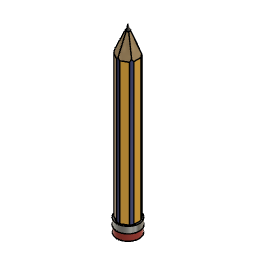
Pencil (Autodesk Fusion 360 design; units mm, degrees)
Autodesk Fusion 360 part; units mm, degrees
sketch "Sketch4" plane through (0, 0, 0) normal (0, 0, 1) x (1, 0, 0)
  line L0 (10, 5.7735) -> (0, 11.547)
  line L1 (0, 11.547) -> (-10, 5.7735)
  line L2 (-10, 5.7735) -> (-10, -5.7735)
  line L3 (-10, -5.7735) -> (0, -11.547)
  line L4 (0, -11.547) -> (10, -5.7735)
  line L5 (10, -5.7735) -> (10, 5.7735)
extrude "Extrude3" add sketch "Sketch4" along normal blind 150
ref_plane "WorkPlane2" through (0, 0, 172) normal (0, 0, 1) x (1, 0, 0)
sketch "Sketch6" plane through (0, 0, 172) normal (0, 0, 1) x (1, 0, 0)
  circle A0 centre (0, 0) radius 2
  constraint coincident A0.centre origin
loft "Loft1" add profiles "Sketch6" section 1 face at (3.3333, 1.9245, 150) section 2
ref_plane "WorkPlane3" through (0, 0, 178) normal (0, 0, 1) x (1, 0, 0)
sketch "Sketch7" plane through (0, 0, 178) normal (0, 0, 1) x (1, 0, 0)
  circle A0 centre (0, 0) radius 0.0005
  dimension "d11" = 0.001
  constraint coincident A0.centre origin
  measures "d11" diameter of A0
loft "Loft2" add section 1 face at (-0.1251, 0.4887, 172) section 2 point at (0, 0, 178)
sketch "Sketch8" plane through (0, 0, 0) normal (0, 0, -1) x (1, 0, 0)
  line L0 (10, -5.7735) -> (10, 5.7735)
  line L1 (10, 5.7735) -> (0, 11.547)
  line L2 (0, 11.547) -> (-10, 5.7735)
  line L3 (-10, 5.7735) -> (-10, -5.7735)
  line L4 (-10, -5.7735) -> (0, -11.547)
  line L5 (0, -11.547) -> (10, -5.7735)
  circle A0 centre (0, 0) radius 12
  constraint coincident A0.centre origin
extrude "Extrude4" add sketch "Sketch8" along normal blind 7 contours L0 L1 L2 L3 L4 L5 | A0
sketch "Sketch9" plane through (0, 0, -7) normal (0, 0, -1) x (1, 0, 0)
  circle A0 centre (0, 0) radius 12
  circle A1 centre (0, 0) radius 11.75
  dimension "d14" = 23.5
  constraint concentric A0 A1
  measures "d14" diameter of A1
extrude "Extrude5" add sketch "Sketch9" along normal blind 7 contours A1
chamfer "Chamfer1" distance 2 angle 45 6 edges at (0, -11.547, 75) (10, -5.7735, 75) (10, 5.7735, 75) (0, 11.547, 75) (-10, 5.7735, 75) (-10, -5.7735, 75)
fillet "Fillet1" radius 0.1 12 edges at (1.7321, -10.547, 75) (8.2679, -6.7735, 75) (10, -3.7735, 75) (10, 3.7735, 75) (8.2679, 6.7735, 75) (1.7321, 10.547, 75) (-1.7321, 10.547, 75) (-8.2679, 6.7735, 75) (-10, 3.7735, 75) (-10, -3.7735, 75) (-8.2679, -6.7735, 75) (-1.7321, -10.547, 75)
